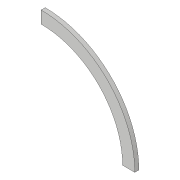
# Autodesk Inventor part: curved_line_sml
Saved by Autodesk Inventor 2018 (Build 220112000, 112)
## iProperties
Created: 2017-08-24
Part Number: curved_line_sml
Material: Generic
Document SubType Name: Modeling
Designer: Platform
Density: 1 g/cm^3
Appearance: Default
Author: Platform
Autodesk Inventor part; units mm, degrees
ref_plane "YZ Plane" through (0, 0, 0) normal (1, 0, 0) x (0, 1, 0)
ref_plane "XZ Plane" through (0, 0, 0) normal (0, 1, 0) x (-1, 0, 0)
ref_plane "XY Plane" through (0, 0, 0) normal (0, 0, 1) x (1, 0, 0)
sketch "Sketch1" plane through (0, 0, 0) normal (0, 0, 1) x (1, 0, 0)
  arc A0 (100, 0) -> (0, 100) centre (0, 0) ccw
  arc A1 (115, 0) -> (0, 115) centre (0, 0) ccw
  line L0 (0, 115) -> (0, 100)
  line L1 (100, 0) -> (115, 0)
  dimension "d0" = 200
  dimension "d1" = 230
  constraints: 4 end point, 4 point on circle, 2 centre point, 2 coincident, 1 horizontal, 1 vertical
  measures "d0" diameter of A0
  measures "d1" diameter of A1
extrude "Extrusion1" add sketch "Sketch1" along normal blind 5
body "Solid1"
